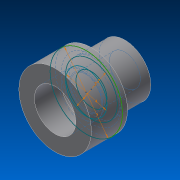
# Autodesk Inventor part: m.2 support
Saved by Autodesk Inventor 2015 (Build 190159000, 159)
## iProperties
Created: 2017-03-26
Part Number: m.2 support
Material: Generic
Document SubType Name: Modeling
Designer: ZigZagJoe
Density: 1 g/cm^3
Appearance: Default
Author: ZigZagJoe
Autodesk Inventor part; units mm, degrees
ref_plane "YZ Plane" through (0, 0, 0) normal (1, 0, 0) x (0, 1, 0)
ref_plane "XZ Plane" through (0, 0, 0) normal (0, 1, 0) x (-1, 0, 0)
ref_plane "XY Plane" through (0, 0, 0) normal (0, 0, 1) x (1, 0, 0)
sketch "Sketch1" plane through (0, 0, 0) normal (0, 1, 0) x (-1, 0, 0)
  circle A0 centre (0, 0) radius 3.5
  circle A1 centre (0, 0) radius 2
  dimension "d0" = 7
  dimension "d2" = 4
  constraints: 2 centre point, 1 coincident
  measures "d0" diameter of A0
  measures "d2" diameter of A1
extrude "Extrusion1" add sketch "Sketch1" against normal blind 3
extrude "Extrusion2" add sketch "Sketch1" along normal blind 0.5 contours A0 | A1
sketch "Sketch2" plane through (0, 0.5, 0) normal (0, 1, 0) x (1, 0, 0)
  circle A0 centre (0, 0) radius 2.5
  circle A1 centre (0, 0) radius 1.5
  dimension "d10" = 5
  dimension "d11" = 3
  constraints: 2 centre point, 2 coincident
  measures "d10" diameter of A0
  measures "d11" diameter of A1
extrude "Extrusion4" add sketch "Sketch2" along normal blind 3.25
fillet "Fillet1" radius 0.4 2 edges at (-2.5, 0.5, 0) (2, 0, 0)
extrude "Extrusion5" cut sketch "Sketch2" against normal blind 3.25 contours A1
body "Solid1"
